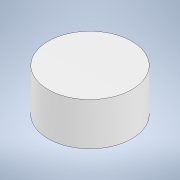
# Autodesk Inventor part: Solid13_mother_m2
Saved by Autodesk Inventor 2020.3 (Build 243373000, 373)
## iProperties
Created: 2021-03-23
Part Number: Solid13_mother_m2
Material: ABS Plastic
Document SubType Name: Modeling
Designer: sanyi
Density: 1.06 g/cm^3
Appearance: Smooth - White
Author: sanyi
Autodesk Inventor part; units mm, degrees
ref_plane "YZ Plane" through (0, 0, 0) normal (1, 0, 0) x (0, 1, 0)
ref_plane "XZ Plane" through (0, 0, 0) normal (0, 1, 0) x (-1, 0, 0)
ref_plane "XY Plane" through (0, 0, 0) normal (0, 0, 1) x (1, 0, 0)
sketch "Sketch1" plane through (0, 0, 0) normal (0, 1, 0) x (-1, 0, 0)
  circle A0 centre (0, 0) radius 2.455
  line L0 (0, -2.455) -> (2.1261, -1.2275)
  line L1 (2.1261, -1.2275) -> (2.1261, 1.2275)
  line L2 (2.1261, 1.2275) -> (0, 2.455)
  line L3 (0, 2.455) -> (-2.1261, 1.2275)
  line L4 (-2.1261, 1.2275) -> (-2.1261, -1.2275)
  line L5 (-2.1261, -1.2275) -> (0, -2.455)
  dimension "d0" = 4.91
  constraints: 12 end point, 6 point on circle, 3 equal length, 2 parallel, 1 centre point, 1 coincident, 1 vertical
  measures "d0" diameter of A0
extrude "Extrusion1" add sketch "Sketch1" along normal blind 2.5
body "Solid1"
